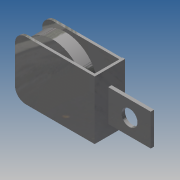
# Autodesk Inventor part: 0pulley
Saved by Autodesk Inventor 2014 SP1 (Build 180222100, 222)
## iProperties
Company: HERA Project
Created: 2013-12-17
Part Number: 0pulley
Material: Steel, Alloy
Document SubType Name: Modeling
Designer: Dave
Density: 7.85 g/cm^3
Mass: 122.938 g
Surface Area: 122.268 cm^2
Volume: 15.6609 cm^3
Description: feed pulley
Appearance: Semi-Polished
Author: David DeBoer
Autodesk Inventor part; units mm, degrees
ref_plane "YZ Plane" through (0, 0, 0) normal (1, 0, 0) x (0, 1, 0)
ref_plane "XZ Plane" through (0, 0, 0) normal (0, 1, 0) x (-1, 0, 0)
sketch "Sketch1" plane through (0, 0, 0) normal (0, 0, 1) x (1, 0, 0)
  circle A0 centre (0, 0) radius 19.05
  dimension "d0" = 38.1
  constraints: 1 centre point, 1 coincident
  measures "d0" diameter of A0
extrude "wheel" add sketch "Sketch1" along normal blind 7.62
sketch "Sketch2" plane through (0, 0, 7.62) normal (0, 0, 1) x (1, 0, 0)
  circle A0 centre (0, 0) radius 19.05 projected
  circle A1 centre (0, 0) radius 3.81
  dimension "d4" = 7.62
  constraints: 1 centre point, 1 coincident
  measures "d4" diameter of A1
extrude "axle" add sketch "Sketch2" along normal blind 5.08 and the other way blind 12.7 contours A1
sketch "Sketch3" plane through (0, 0, 12.7) normal (0, 0, 1) x (1, 0, 0)
  line L0 (-11.1125, -17.4625) -> (28.575, -17.4625)
  line L1 (28.575, -17.4625) -> (28.575, 17.4625)
  line L2 (28.575, 17.4625) -> (-11.1125, 17.4625)
  line L3 (-17.4625, 11.1125) -> (-17.4625, -11.1125)
  arc A0 (-11.1125, 17.4625) -> (-17.4625, 11.1125) centre (-11.1125, 11.1125) ccw
  arc A1 (-17.4625, -11.1125) -> (-11.1125, -17.4625) centre (-11.1125, -11.1125) ccw
  point P0 (-17.4625, -17.4625)
  point P1 (-17.4625, 17.4625)
  dimension "d13" = 6.35
  constraints: 8 end point, 4 point on circle, 4 point on line, 4 tangent, 2 centre point, 2 parallel, 1 equal radius, 1 horizontal, 1 perpendicular
  measures "d13" radius of A0
extrude "side" add sketch "Sketch3" against normal blind 1.524
ref_plane "Work Plane1" through (0, 0, 3.81) normal (0, 0, -1) x (-1, 0, 0)
mirror "Mirror1" about plane through (0, 0, 3.81) normal (0, 0, -1) of "side"
sketch "Sketch4" plane through (28.575, -17.4625, 12.7) normal (1, 0, 0) x (0, 0, -1)
  line L0 (0, 0) -> (18.1871, 0)
  line L1 (18.1871, 0) -> (18.1871, 34.925)
  line L2 (18.1871, 34.925) -> (0, 34.925)
  line L3 (0, 34.925) -> (0, 0)
  point P0 (12.7, 17.4625)
  constraints: 8 end point, 2 parallel, 1 horizontal, 1 perpendicular
extrude "Extrusion4" add sketch "Sketch4" along normal blind 1.524
sketch "Sketch5" plane through (30.099, -17.4625, 12.7) normal (1, 0, 0) x (0, 0, -1)
  line L0 (0, 0) -> (18.1871, 0) projected
  line L1 (18.1871, 34.925) -> (0, 34.925) projected
  line L2 (8.0841, 6.35) -> (10.103, 6.35)
  line L3 (10.103, 6.35) -> (10.103, 25.4)
  line L4 (10.103, 25.4) -> (8.0841, 25.4)
  line L5 (8.0841, 25.4) -> (8.0841, 6.35)
  line L6 (9.0935, 34.925) -> (9.0935, 0) construction
  line L7 (9.0935, 25.4) -> (9.0935, 6.35) construction
  point P0 (12.7, 17.4625)
  constraints: 12 end point, 4 midpoint, 2 parallel, 1 collinear, 1 horizontal, 1 perpendicular
extrude "Extrusion5" add sketch "Sketch5" along normal blind 25.4
sketch "Sketch6" plane through (30.099, -11.1125, 4.6159) normal (0, 0, 1) x (1, 0, 0)
  line L0 (25.4, 19.05) -> (25.4, 0) projected
  circle A0 centre (12.7, 9.525) radius 4.7625
  point P0 (-30.099, 11.1125)
  dimension "d19" = 12.7
  constraints: 1 centre point
  measures "d19" distance from line of A0.centre L0
extrude "Extrusion6" cut sketch "Sketch6" against normal blind 25.4
body "Solid1"
